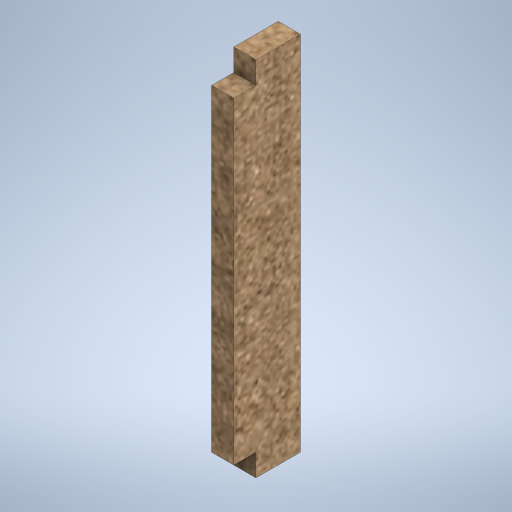
# Autodesk Inventor part: Case_Base3
Saved by Autodesk Inventor 2024 (Build 280153000, 153)
## iProperties
Created: 2023-11-23
Part Number: Case_Base3
Material: MDF Tablero de fibras de densidad media
Document SubType Name: Modeling
Designer: marco
Density: 0.8 g/cm^3
Appearance: Cartón - Ondulado
Author: marco
Autodesk Inventor part; units mm, degrees
ref_plane "YZ Plane" through (0, 0, 0) normal (1, 0, 0) x (0, 1, 0)
ref_plane "XZ Plane" through (0, 0, 0) normal (0, 1, 0) x (-1, 0, 0)
ref_plane "XY Plane" through (0, 0, 0) normal (0, 0, 1) x (1, 0, 0)
sketch "Boceto1" plane through (0, 0, 0) normal (1, 0, 0) x (0, 1, 0)
  line L0 (21.5, 1.5) -> (21.5, 4.5)
  line L1 (24.5, 1.5) -> (21.5, 1.5)
  line L2 (24.5, -4.5) -> (24.5, 1.5)
  line L3 (21.5, -4.5) -> (24.5, -4.5)
  line L4 (-21.5, -4.5) -> (21.5, -4.5)
  line L5 (-24.5, -4.5) -> (-21.5, -4.5)
  line L6 (-24.5, 1.5) -> (-24.5, -4.5)
  line L7 (-21.5, 1.5) -> (-24.5, 1.5)
  line L8 (-21.5, 4.5) -> (-21.5, 1.5)
  line L9 (21.5, 4.5) -> (-21.5, 4.5)
  point P0 (0, 0)
  constraints: 20 end point
extrude "Extrusión1" add sketch "Boceto1" along normal blind 3
